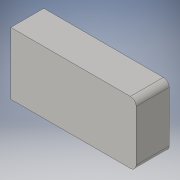
# Autodesk Inventor part: Aidan Sherry Battery Pack
Saved by Autodesk Inventor 2016 (Build 200138000, 138)
## iProperties
Created: 2016-10-05
Part Number: Aidan Sherry Battery Pack
Material: Generic
Document SubType Name: Modeling
Designer: sherra
Density: 1 g/cm^3
Appearance: Default
Author: sherra
Autodesk Inventor part; units mm, degrees
ref_plane "YZ Plane" through (0, 0, 0) normal (1, 0, 0) x (0, 1, 0)
ref_plane "XZ Plane" through (0, 0, 0) normal (0, 1, 0) x (-1, 0, 0)
ref_plane "XY Plane" through (0, 0, 0) normal (0, 0, 1) x (1, 0, 0)
sketch "Sketch1" plane through (0, 0, 0) normal (0, 0, 1) x (1, 0, 0)
  line L0 (-29.7451, 24.9779) -> (38.6825, 24.9779)
  line L1 (38.6825, 24.9779) -> (38.6825, -9.0073)
  line L2 (38.6825, -9.0073) -> (-29.7451, -9.0073)
  line L3 (-29.7451, -9.0073) -> (-29.7451, 24.9779)
  point P0 (0, 0)
  dimension "d0" = 68.4276
  dimension "d1" = 33.9852
  constraints: 8 end point, 2 parallel, 1 horizontal, 1 perpendicular
  measures "d0" distance of L1.end L2.end
  measures "d1" distance of L2.end L0.start
extrude "Extrusion1" add sketch "Sketch1" along normal blind 18.034
fillet "Fillet1" radius 3.175 1 edges at (38.6825, 24.9779, 9.017)
fillet "Fillet2" radius 3.175 1 edges at (38.6825, -9.0073, 9.017)
body "Solid1"
